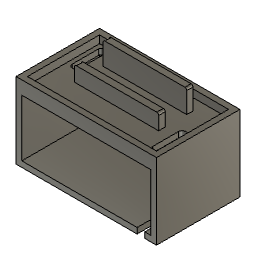
cable_box (Autodesk Fusion 360 design; units mm, degrees)
Autodesk Fusion 360 part; units mm, degrees
sketch "Sketch4" plane through (0, 0, 0) normal (0, 0, 1) x (1, 0, 0)
  line L0 (0, 0) -> (-370, 0)
  line L1 (-370, 0) -> (-370, 220.0001)
  line L2 (-370, 220.0001) -> (0, 220.0001)
  line L3 (0, 220.0001) -> (0, 0)
  constraint horizontal L0
  constraint vertical L1
  constraint horizontal L2
  constraint vertical L3
  constraint coincident L0.start L3.end
extrude "Extrude1" add sketch "Sketch4" along normal blind 180
shell "Shell1" thickness 15 removed faces 1 at (-123.3333, 0, 60)
sketch "Sketch5" plane through (0, 0, 15) normal (0, 0, 1) x (-1, 0, 0)
  line L0 (15, -205.0001) -> (355, -205.0001)
  line L1 (355, -205.0001) -> (355, 0)
  line L2 (355, 0) -> (15, 0)
  line L3 (15, 0) -> (15, -205.0001)
  arc A0 (91.5155, -197.8612) -> (90.4492, -197.9194) centre (90.9821, -197.8846) ccw
sketch "Sketch6" plane through (0, 0, 0) normal (0, 0, 1) x (1, 0, 0)
  line L0 (-30.8887, -0.5052) -> (-30.8887, 189.4948)
  arc A0 (-30.8887, 189.4948) -> (-50.8736, 189.4948) centre (-40.8811, 189.4948) ccw
  line L1 (-50.8736, 189.4948) -> (-50.8736, -0.4766)
  line L2 (-50.8736, -0.4766) -> (-30.8887, -0.5052)
  dimension "d5" = 190
  constraint vertical L0
  constraint tangent L0 A0
  constraint tangent A0 L1
  constraint vertical L1
  measures "d5" distance of L0.start L0.end
extrude "Extrude2" cut sketch "Sketch6" along normal blind 20
sketch "Sketch7" plane through (0, 0, 180) normal (0, 0, 1) x (-1, 0, 0)
  line L0 (0, -220.0001) -> (370, -220.0001)
  line L1 (370, -220.0001) -> (370, 0)
  line L2 (370, 0) -> (0, 0)
  line L3 (0, 0) -> (0, -220.0001)
  line L4 (0, 0) -> (370, 0)
  line L5 (370, 0) -> (370, -220.0001)
  line L6 (370, -220.0001) -> (0, -220.0001)
  line L7 (0, -220.0001) -> (0, 0)
  constraint horizontal L4
  constraint vertical L5
  constraint horizontal L6
  constraint vertical L7
  constraint coincident L0.end L1.start
  constraint coincident L2.end L3.start
extrude "Extrude3" add sketch "Sketch7" along normal blind 20
shell "Shell2" thickness 15 removed faces 1 at (-123.3333, 73.3334, 200)
sketch "cable2" plane through (0, 0, 180) normal (0, 0, 1) x (-1, 0, 0)
  line L0 (15, -205.0001) -> (355, -205.0001)
  line L1 (355, -205.0001) -> (355, -15)
  line L2 (355, -15) -> (15, -15)
  line L3 (15, -15) -> (15, -205.0001)
  line L4 (30.7104, -40.8015) -> (30.7104, -108.2698)
  arc A0 (30.7104, -108.2698) -> (50.329, -108.2698) centre (40.5197, -108.2698) ccw
  line L5 (50.329, -108.2698) -> (50.329, -40.4606)
  arc A1 (50.329, -40.4606) -> (30.7104, -40.8015) centre (40.5168, -40.4606) ccw
  constraint vertical L4
  constraint tangent L4 A0
  constraint tangent A0 L5
  constraint parallel L4 L5
  constraint tangent L5 A1
extrude "Extrude4" cut sketch "cable2" against normal blind 20 contours L4 A0 L5 A1
sketch "cable" plane through (0, 0, 180) normal (0, 0, 1) x (-1, 0, 0)
  line L0 (30.7104, -108.2698) -> (30.7104, -40.8015)
  arc A0 (50.329, -40.4606) -> (30.7104, -40.8015) centre (40.5168, -40.4606) ccw
  line L1 (50.329, -40.4606) -> (50.329, -108.2698)
  arc A1 (30.7104, -108.2698) -> (50.329, -108.2698) centre (40.5197, -108.2698) ccw
  line L2 (15, -205.0001) -> (355, -205.0001)
  line L3 (355, -205.0001) -> (355, -15)
  line L4 (355, -15) -> (15, -15)
  line L5 (15, -15) -> (15, -205.0001)
  line L6 (344.3489, -192.4024) -> (344.3489, -122.5556)
  arc A2 (344.3489, -122.5556) -> (324.7501, -122.5556) centre (334.5495, -122.5556) ccw
  line L7 (324.7501, -122.5556) -> (324.7501, -189.3593)
  arc A3 (324.7501, -189.3593) -> (344.3489, -192.4024) centre (334.7857, -189.3593) ccw
  constraint parallel L3 L6
  constraint tangent L6 A2
  constraint tangent A2 L7
  constraint parallel L6 L7
  constraint tangent L7 A3
extrude "Extrude5" cut sketch "cable" against normal blind 20 contours L6 A2 L7 A3
sketch "wedge big" plane through (0, 0, 180) normal (0, 0, 1) x (-1, 0, 0)
  line L0 (344.3489, -122.5556) -> (344.3489, -192.4024)
  arc A0 (324.7501, -189.3593) -> (344.3489, -192.4024) centre (334.7857, -189.3593) ccw
  line L1 (324.7501, -189.3593) -> (324.7501, -122.5556)
  arc A1 (344.3489, -122.5556) -> (324.7501, -122.5556) centre (334.5495, -122.5556) ccw
  line L2 (30.7104, -108.2698) -> (30.7104, -40.8015)
  arc A2 (50.329, -40.4606) -> (30.7104, -40.8015) centre (40.5168, -40.4606) ccw
  line L3 (50.329, -40.4606) -> (50.329, -108.2698)
  arc A3 (30.7104, -108.2698) -> (50.329, -108.2698) centre (40.5197, -108.2698) ccw
  line L4 (15, -205.0001) -> (355, -205.0001)
  line L5 (355, -205.0001) -> (355, -15)
  line L6 (355, -15) -> (15, -15)
  line L7 (15, -15) -> (15, -205.0001)
  line L8 (298.854, -174.169) -> (78.0156, -174.169)
  line L9 (78.0156, -174.169) -> (78.0156, -158.01)
  line L10 (78.0156, -158.01) -> (298.854, -158.01)
  line L11 (298.854, -158.01) -> (298.854, -174.169)
  constraint horizontal L8
  constraint vertical L9
  constraint horizontal L10
  constraint vertical L11
extrude "Extrude6" add sketch "wedge big" along normal blind 40 contours L8 L9 L10 L11
sketch "wedge small" plane through (0, 0, 180) normal (0, 0, 1) x (-1, 0, 0)
  line L0 (298.854, -158.01) -> (298.854, -174.169)
  line L1 (298.854, -174.169) -> (78.0156, -174.169)
  line L2 (78.0156, -174.169) -> (78.0156, -158.01)
  line L3 (78.0156, -158.01) -> (298.854, -158.01)
  line L4 (344.3489, -122.5556) -> (344.3489, -192.4024)
  arc A0 (324.7501, -189.3593) -> (344.3489, -192.4024) centre (334.7857, -189.3593) ccw
  line L5 (324.7501, -189.3593) -> (324.7501, -122.5556)
  arc A1 (344.3489, -122.5556) -> (324.7501, -122.5556) centre (334.5495, -122.5556) ccw
  line L6 (30.7104, -108.2698) -> (30.7104, -40.8015)
  arc A2 (50.329, -40.4606) -> (30.7104, -40.8015) centre (40.5168, -40.4606) ccw
  line L7 (50.329, -40.4606) -> (50.329, -108.2698)
  arc A3 (30.7104, -108.2698) -> (50.329, -108.2698) centre (40.5197, -108.2698) ccw
  line L8 (15, -205.0001) -> (355, -205.0001)
  line L9 (355, -205.0001) -> (355, -15)
  line L10 (355, -15) -> (15, -15)
  line L11 (15, -15) -> (15, -205.0001)
  line L12 (300.118, -101.3077) -> (78.2153, -101.3077)
  line L13 (78.2153, -101.3077) -> (78.2153, -83.9988)
  line L14 (78.2153, -83.9988) -> (300.118, -83.9988)
  line L15 (300.118, -83.9988) -> (300.118, -101.3077)
  constraint horizontal L12
  constraint vertical L13
  constraint horizontal L14
  constraint vertical L15
extrude "Extrude7" add sketch "wedge small" along normal blind 40 contours L12 L13 L14 L15
extrude "Extrude8" add 1 faces at (-225.2412, 168.7826, 220) along direction (0, 0, 1) blind 40
extrude "Extrude9" cut 1 faces at (-225.2412, 168.7826, 260) along direction (0, 0, -1) blind 20
fillet "Fillet7" radius 5 2 edges at (-298.854, 166.0895, 240) (-78.0156, 166.0895, 240)
fillet "Fillet8" radius 5 2 edges at (-300.118, 92.6532, 220) (-78.2153, 92.6532, 220)
fillet "Fillet9" [rolled back] radius 10
